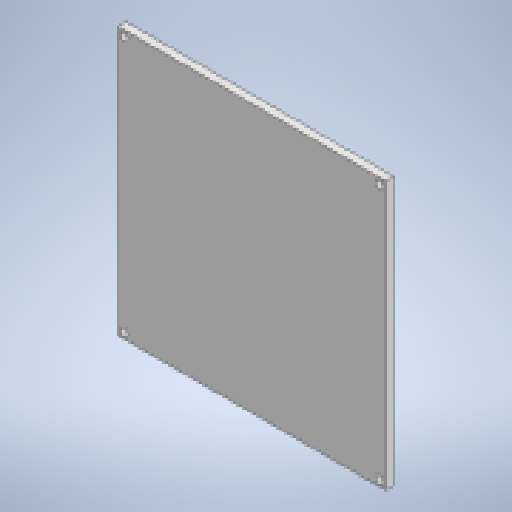
# Autodesk Inventor part: Disco_Superior
Saved by Autodesk Inventor 2024 (Build 280153000, 153)
## iProperties
Created: 2025-02-27
Part Number: Disco_Superior
Material: Genérico
Document SubType Name: Modeling
Designer: sergi
Density: 1 g/cm^3
Appearance: Valor por defecto
Author: sergi
Autodesk Inventor part; units mm, degrees
ref_plane "YZ Plane" through (0, 0, 0) normal (1, 0, 0) x (0, 1, 0)
ref_plane "XZ Plane" through (0, 0, 0) normal (0, 1, 0) x (-1, 0, 0)
ref_plane "XY Plane" through (0, 0, 0) normal (0, 0, 1) x (1, 0, 0)
sketch "Boceto1" plane through (0, 0, 0) normal (0, 0, 1) x (1, 0, 0)
  line L0 (30, -30) -> (-33, -30) projected
  line L1 (-33, -30) -> (-33, -33) projected
  line L2 (-33, -33) -> (33, -33) projected
  line L3 (33, -33) -> (33, 33) projected
  line L4 (33, 33) -> (-33, 33) projected
  line L5 (-33, 33) -> (-33, 30) projected
  line L6 (-33, 30) -> (30, 30) projected
  line L7 (30, 30) -> (30, -30) projected
  line L8 (-33, 33) -> (33, 33)
  line L9 (33, 33) -> (33, -33)
  line L10 (33, -33) -> (-33, -33)
  line L11 (-33, -33) -> (-33, 33)
  point P0 (0, 0)
  constraints: 8 end point, 2 parallel, 1 horizontal, 1 perpendicular
extrude "Extrusión1" add sketch "Boceto1" along normal blind 2
